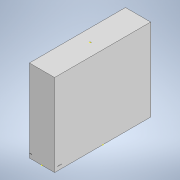
# Autodesk Inventor part: wheelchair_box_retracted
Saved by Autodesk Inventor 2021 (Build 250183000, 183)
## iProperties
Created: 2021-05-27
Part Number: wheelchair_box_retracted
Material: Generic
Document SubType Name: Modeling
Designer: Watchdog
Density: 1 g/cm^3
Appearance: Default
Author: Watchdog
Autodesk Inventor part; units mm, degrees
ref_plane "YZ Plane" through (0, 0, 0) normal (1, 0, 0) x (0, 1, 0)
ref_plane "XZ Plane" through (0, 0, 0) normal (0, 1, 0) x (-1, 0, 0)
ref_plane "XY Plane" through (0, 0, 0) normal (0, 0, 1) x (1, 0, 0)
sketch "Sketch1" plane through (0, 0, 0) normal (0, 1, 0) x (-1, 0, 0)
  line L0 (140, -533.5) -> (-140, -533.5)
  line L1 (-140, -533.5) -> (-140, 533.5)
  line L2 (-140, 533.5) -> (140, 533.5)
  line L3 (140, 533.5) -> (140, -533.5)
  point P0 (0, 0)
  dimension "d0" = 280
  dimension "d1" = 1067
  dimension "d2" = 533.5
  dimension "d3" = 140
  constraints: 8 end point, 2 parallel, 1 horizontal, 1 perpendicular
  measures "d0" distance of L0.start L0.end
  measures "d1" distance of L0.end L1.end
  measures "d2" distance from line of point (0, 0) L0
  measures "d3" distance from line of point (0, 0) L3
extrude "Extrusion1" add sketch "Sketch1" along normal blind 914
sketch "Sketch2" plane through (-140, 0, 533.5) normal (0, 0, 1) x (1, 0, 0)
  line L0 (-0.7301, 50.1324) -> (28.3017, 50.1324) construction
  line L1 (28.3017, 50.1324) -> (28.3017, 43.7754) construction
  line L2 (28.3017, 43.7754) -> (-0.7301, 43.7754) construction
  line L3 (-0.7301, 43.7754) -> (-0.7301, 50.1324) construction
  point P0 (140, 0)
  constraints: 2 other
sketch "Sketch3" plane through (-140, 0, -533.5) normal (-1, 0, 0) x (0, 0, 1)
  line L0 (30.8104, 48.5767) -> (82.087, 48.5767) construction
  line L1 (82.087, 48.5767) -> (82.087, 42.2296) construction
  line L2 (82.087, 42.2296) -> (30.8104, 42.2296) construction
  line L3 (30.8104, 42.2296) -> (30.8104, 48.5767) construction
  point P0 (533.5, 0)
  constraints: 2 other
sketch "Sketch4" plane through (140, 0, 533.5) normal (1, 0, 0) x (0, 0, -1)
  line L0 (32.5592, 45.8564) -> (78.0917, 45.8564) construction
  line L1 (78.0917, 45.8564) -> (78.0917, 29.6042) construction
  line L2 (78.0917, 29.6042) -> (32.5592, 29.6042) construction
  line L3 (32.5592, 29.6042) -> (32.5592, 45.8564) construction
  point P0 (533.5, 0)
  constraints: 2 other
sketch "Sketch5" plane through (140, 0, -533.5) normal (0, 0, -1) x (-1, 0, 0)
  line L0 (-10.0202, 53.8243) -> (35.5122, 53.8243) construction
  line L1 (35.5122, 53.8243) -> (35.5122, 37.5621) construction
  line L2 (35.5122, 37.5621) -> (-10.0202, 37.5621) construction
  line L3 (-10.0202, 37.5621) -> (-10.0202, 53.8243) construction
  point P0 (140, 0)
  constraints: 2 other
sketch "Sketch6" plane through (0, 914, 0) normal (0, 1, 0) x (1, 0, 0)
  line L0 (-31.9661, 8.1609) -> (33.1319, 8.1609) construction
  line L1 (33.1319, 8.1609) -> (33.1319, 1.8038) construction
  line L2 (33.1319, 1.8038) -> (-31.9661, 1.8038) construction
  line L3 (-31.9661, 1.8038) -> (-31.9661, 8.1609) construction
  point P0 (0, 0)
  constraints: 2 other
sketch "Sketch7" plane through (0, 0, 0) normal (0, -1, 0) x (1, 0, 0)
  line L0 (2.9613, 16.4046) -> (2.9613, -29.1279) construction
  line L1 (2.9613, -29.1279) -> (-13.3107, -29.1279) construction
  line L2 (-13.3107, -29.1279) -> (-13.3107, 16.4046) construction
  line L3 (-13.3107, 16.4046) -> (2.9613, 16.4046) construction
  point P0 (0, 0)
  constraints: 2 other
equation "\"d0\" = y"
equation "\"d1\" = x"
equation "\"d2\" = 0.5 * d1"
equation "\"d3\" = 0.5 * d0"
equation "\"d4\" = z"
equation "\"x\" = wheelchair_deployed_length"
equation "\"y\" = wheelchair_folded_width"
equation "\"z\" = wheelchair_deployed_height"
equation "\"hoop_angle_z\" = 45deg"
equation "\"hoop_bearing_length\" = 5deg"
equation "\"hoop_cable_diam\" = 5"
equation "\"hoop_cable_pulley_diam\" = 22"
equation "\"rack_tooth_addendum\" = 5"
equation "\"rack_tooth_dedendum\" = 5"
equation "\"rack_tooth_thickness\" = 5"
equation "\"secure_arm_angle\" = 20deg"
equation "\"secure_arm_hold_length\" = 35"
equation "\"secure_arm_radii\" = 9"
equation "\"support_baseClamp_platformLengthBuffer\" = 35"
equation "\"support_baseClamp_platformThickness\" = 15"
equation "\"support_baseClamp_platformWidthBuffer\" = 0"
equation "\"support_baseClamp_sleeveHoleDiameter\" = 12"
equation "\"support_baseClamp_sleeveSweepTerminationAngle\" = 55deg"
equation "\"support_baseClamp_thickness\" = 8"
equation "\"support_frame_endHoleBuffer\" = 25"
equation "\"support_frame_squareBarFillet\" = 2"
equation "\"support_frame_squareBarThickness\" = 5"
equation "\"hoop_tabs_thickness\" = 6"
equation "\"hoop_tabs_hole\" = 4"
equation "\"wheelchair_deployed_width\" = 635"
equation "\"wheelchair_deployed_length\" = 1067"
equation "\"wheelchair_deployed_height\" = 914"
equation "\"wheelchair_folded_width\" = 280"
body "Solid1"
